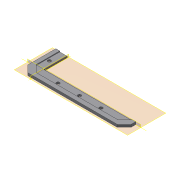
# Autodesk Inventor part: Cycl_soportePCB_B
Saved by Autodesk Inventor 2015 SP2 (Build 190223200, 223)
## iProperties
Created: 2015-04-21
Material: Genérico
Document SubType Name: Modeling
Designer: E.Beroiz
Density: 1 g/cm^3
Appearance: Valor por defecto
Description: Cycl_soportePCB_B
Author: E.Beroiz
Autodesk Inventor part; units mm, degrees
sketch "Boceto1" plane through (0, 0, 0) normal (0, 0, 1) x (1, 0, 0)
  line L0 (0, 0) -> (107.005, 0)
  line L1 (107.005, 0) -> (107.005, -5.5)
  line L2 (107.005, -5.5) -> (99.0087, -13.4963)
  line L3 (99.0087, -13.4963) -> (-4.9913, -13.4963)
  line L4 (-4.9913, -13.4963) -> (-12.9876, -5.5)
  line L5 (-12.9876, -5.5) -> (-12.9876, 27)
  line L6 (-12.9876, 27) -> (0, 27)
  line L7 (0, 27) -> (0, 0)
  line L8 (107.0124, -0.0005) -> (107.0124, -5.5005) projected
  line L9 (107.0124, -5.5005) -> (82.0124, -30.5) projected
  dimension "d0" = 107.005
  dimension "d1" = 5.5
  dimension "d5" = 32.5
  dimension "d8" = 27
  dimension "d34" = 135
  constraints: 16 end point, 3 perpendicular, 2 vertical, 1 horizontal, 1 parallel
  measures "d0" distance of L0.start L0.end
  measures "d1" distance of L0.end L1.end
  measures "d5" distance of L4.end L5.end
  measures "d8" distance of L6.end L0.start
  measures "d34" angle of L1 L2
extrude "Extrusión1" add sketch "Boceto1" along normal blind 3
sketch "Boceto2" plane through (0, 0, 3) normal (0, 0, 1) x (1, 0, 0)
  circle A0 centre (-5.5, 12) radius 1.89
  line L0 (0, 27) -> (-12.9876, 27) projected
  point P0 (0, 0)
  dimension "d11" = 3.78
  dimension "d12" = 15
  dimension "d13" = 5.5
  constraints: 1 centre point
  measures "d11" diameter of A0
  measures "d12" distance from line of L0 A0.centre
  measures "d13" horizontal distance of L0.start A0.centre
extrude "Extrusión2" cut sketch "Boceto2" against normal through all
sketch "Boceto3" plane through (0, 0, 3) normal (0, 0, 1) x (1, 0, 0)
  circle A0 centre (22.0124, -5.5) radius 1.89
  line L0 (-12.9876, 27) -> (-12.9876, -5.5) projected
  point P0 (0, 0)
  dimension "d16" = 3.78
  dimension "d17" = 5.5
  dimension "d18" = 35
  constraints: 1 centre point
  measures "d16" diameter of A0
  measures "d17" vertical distance of A0.centre point (0, 0)
  measures "d18" distance from line of L0 A0.centre
extrude "Extrusión3" cut sketch "Boceto3" against normal through all
pattern_linear "Patrón rectangular1" count 3 spacing 25 along (1, 0, 0) of "Extrusión3"
sketch "Boceto4" plane through (0, 0, 3) normal (0, 0, 1) x (1, 0, 0)
  line L0 (0, 0) -> (0, 27) projected
  line L1 (107.005, 0) -> (0, 0) projected
  line L2 (0, 27) -> (-8.5, 27)
  line L3 (0, 27) -> (-12.9876, 27) projected
  line L4 (-8.5, 27) -> (-8.5, -0.4998)
  line L5 (-0.4998, -8.5) -> (94.505, -8.5)
  line L6 (94.505, -8.5) -> (102.505, -1)
  line L7 (102.505, -1) -> (102.505, 0)
  line L8 (-8.5, -0.4998) -> (-0.4998, -8.5)
  line L9 (107.005, -5.5) -> (107.005, 0) projected
  dimension "d24" = 8.5
  dimension "d25" = 8.5
  dimension "d26" = 135
  dimension "d27" = 11.314
  dimension "d28" = 1
  dimension "d30" = 12.5
  dimension "d31" = 4.5
  constraints: 12 end point, 2 perpendicular, 2 point on line, 1 vertical
  measures "d24" distance of L0.end L2.end
  measures "d25" distance between parallel lines of L1 L5
  measures "d26" angle of L5 L8
  measures "d27" distance of L4.end L5.start
  measures "d28" distance of L6.end L7.end
  measures "d30" distance from line of L9 L5.end
  measures "d31" distance between parallel lines of L9 L7
extrude "Extrusión4" cut sketch "Boceto4" against normal blind 1
